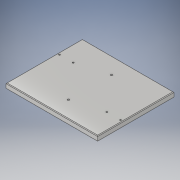
# Autodesk Inventor part: Bodenplatte
Saved by Autodesk Inventor 2019 (Build 230136000, 136)
## iProperties
Created: 2018-09-19
Part Number: Bodenplatte
Material: Generisch
Document SubType Name: Modeling
Designer: nico-
Density: 1 g/cm^3
Appearance: Aluminium - poliert
Author: nico-
Autodesk Inventor part; units mm, degrees
ref_plane "YZ Plane" through (0, 0, 0) normal (1, 0, 0) x (0, 1, 0)
ref_plane "XZ Plane" through (0, 0, 0) normal (0, 1, 0) x (-1, 0, 0)
ref_plane "XY Plane" through (0, 0, 0) normal (0, 0, 1) x (1, 0, 0)
sketch "Skizze2" plane through (0, 0, 0) normal (0, 1, 0) x (-1, 0, 0)
  line L0 (150, 125) -> (-150, 125)
  line L1 (-150, 125) -> (-150, -125)
  line L2 (-150, -125) -> (150, -125)
  line L3 (150, -125) -> (150, 125)
  point P0 (0, 0)
  dimension "d0" = 300
  dimension "d1" = 250
  dimension "d6" = 125
  dimension "d7" = 150
  constraints: 8 end point, 2 parallel, 1 horizontal, 1 perpendicular
  measures "d0" distance of L2.end L1.end
  measures "d1" distance of L1.end L0.end
  measures "d6" distance from line of point (0, 0) L2
  measures "d7" distance from line of point (0, 0) L3
extrude "Extrusion1" add sketch "Skizze2" along normal blind 15
sketch "Skizze3" plane through (0, 15, 0) normal (0, 1, 0) x (1, 0, 0)
  circle A0 centre (0, -70.5) radius 3.25
  circle A1 centre (0, 70.5) radius 3.25
  point P0 (0, 0)
  dimension "d8" = 6.5
  dimension "d9" = 6.5
  dimension "d16" = 70.5
  dimension "d17" = 70.5
  constraints: 2 centre point
  measures "d8" diameter of A0
  measures "d9" diameter of A1
  measures "d16" distance of point (0, 0) A0.centre
  measures "d17" distance of point (0, 0) A1.centre
extrude "Extrusion2" cut sketch "Skizze3" against normal blind 15
sketch "Skizze4" plane through (0, 0, 0) normal (0, -1, 0) x (1, 0, 0)
  circle A0 centre (0, 70.5) radius 6.5
  circle A1 centre (0, -70.5) radius 6.5
  point P0 (0, 0)
  dimension "d12" = 13
  dimension "d13" = 13
  dimension "d18" = 70.5
  dimension "d19" = 70.5
  constraints: 2 centre point
  measures "d12" diameter of A0
  measures "d13" diameter of A1
  measures "d18" distance of point (0, 0) A0.centre
  measures "d19" distance of point (0, 0) A1.centre
extrude "Extrusion3" cut sketch "Skizze4" against normal blind 7
chamfer "Fase1" distance 2 angle 45 4 edges at (0, 15, 125) (150, 15, 0) (0, 15, -125) (-150, 15, 0)
sketch "Skizze5" plane through (0, 15, 0) normal (0, 1, 0) x (1, 0, 0)
  circle A0 centre (142.5, -42.5) radius 2.5
  circle A1 centre (97.5, -42.5) radius 2.5
  circle A2 centre (-142.5, 42.5) radius 2.5
  circle A3 centre (-97.5, 42.5) radius 2.5
  point P0 (0, 0)
  dimension "d23" = 5
  dimension "d24" = 5
  dimension "d25" = 5
  dimension "d26" = 5
  constraints: 4 centre point
  measures "d23" diameter of A0
  measures "d24" diameter of A1
  measures "d25" diameter of A2
  measures "d26" diameter of A3
extrude "Extrusion4" cut sketch "Skizze5" against normal blind 20
thread "Gewinde1" size "M5x0.8" class "6H" standard "ANSI Metric M Profile" full length
thread "Gewinde2" size "M5x0.8" class "6H" standard "ANSI Metric M Profile" full length
thread "Gewinde3" size "M5x0.8" class "6H" standard "ANSI Metric M Profile" full length
thread "Gewinde4" size "M5x0.8" class "6H" standard "ANSI Metric M Profile" full length
